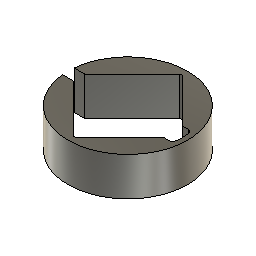
6_tube_notcher_spacer (Autodesk Fusion 360 design; units mm, degrees)
Autodesk Fusion 360 part; units mm, degrees
sketch "Sketch1" plane through (0, 0, 0) normal (0, 0, 1) x (1, 0, 0)
  line L0 (0.7071, 27.5772) -> (23.2843, 5)
  line L1 (23.2843, -5) -> (0.7071, -27.5772)
  line L2 (-0.7071, -27.5772) -> (-25.2843, -3)
  line L3 (-25.2843, 3) -> (-0.7071, 27.5772)
  line L4 (0, 0) -> (57.5603, 0) construction
  line L5 (31, 0) -> (31, -17.1775)
  line L6 (-25.2843, 3) -> (-30.8545, 3)
  line L7 (-25.2843, -3) -> (-30.8545, -3)
  arc A0 (0.7071, 27.5772) -> (-0.7071, 27.5772) centre (0, 26.8701) ccw
  arc A1 (-0.7071, -27.5772) -> (0.7071, -27.5772) centre (0, -26.8701) ccw
  arc A2 (-30.8545, -3) -> (-30.8545, 3) centre (0, 0) ccw
  line L8 (26.2897, 5) -> (23.2843, 5)
  line L9 (26.2897, -5) -> (23.2843, -5)
  arc A3 (28.2701, -3.2791) -> (28.2701, 3.2791) centre (5, 0) ccw
  arc A4 (28.2701, 3.2791) -> (26.2897, 5) centre (26.2897, 3) ccw
  arc A5 (26.2897, -5) -> (28.2701, -3.2791) centre (26.2897, -3) ccw
  point P0 (0, 28.2843)
  point P1 (28.2843, 0)
  point P2 (29, 5)
  dimension "d1" = 62
  dimension "d2" = 40
  dimension "d4" = 20
  dimension "d5" = 20
  dimension "d7" = 45
  dimension "d9" = 3
  dimension "d11" = 1
  dimension "d13" = 5
  dimension "d14" = 5
  dimension "d15" = 47
  dimension "d16" = 2
  constraint coincident L4.start A2.centre
  constraint perpendicular L0 L3
  constraint perpendicular L0 L1
  constraint perpendicular L1 L2
  constraint horizontal L4
  constraint coincident L5.start A2
  constraint coincident L4 L5.start
  constraint tangent L5 A2
  constraint horizontal L6
  constraint symmetric L4 L3.start L2.end
  constraint symmetric L4 L6.end L7.end
  constraint coincident P0 L0
  constraint coincident P0 L3
  constraint tangent L0 A0
  constraint tangent L3 A0
  constraint coincident P1 L0
  constraint coincident P1 L1
  constraint tangent L1 A1
  constraint tangent L2 A1
  constraint equal A0 A1
  constraint coincident L4 A3.centre
  constraint horizontal L8
  constraint tangent A3 A4
  constraint tangent L8 A4
  constraint tangent A3 A5
  constraint tangent L9 A5
  constraint equal A4 A5
  measures "d1" diameter of A2
  measures "d2" distance of P0 P1
  measures "d4" distance of L4.start L3
  measures "d5" distance of L4.start L0
  measures "d7" angle of L1 L4
  measures "d9" distance of L4.start L6
  measures "d11" radius of A0
  measures "d13" distance of L4 L8
  measures "d14" distance of L4.start A3.centre
  measures "d15" diameter of A3
  measures "d16" radius of A4
extrude "Extrude1" add sketch "Sketch1" along normal blind 20
